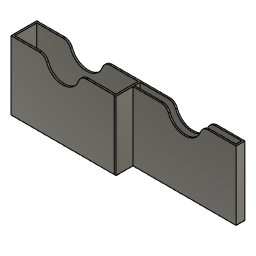
Food_Chain_Magnate_Reserve_CEO v1 (Autodesk Fusion 360 design; units mm, degrees)
Autodesk Fusion 360 part; units mm, degrees
sketch "Sketch1" plane through (0, 0, 0) normal (0, 0, 1) x (1, 0, 0)
  line L0 (-48.6499, 24.8) -> (41.3501, 24.8)
  line L1 (40, 23.2) -> (40, 3.6)
  line L2 (40, 2) -> (-51.6764, 2)
  line L3 (-50, 3.6) -> (-50, 23.2)
  line L4 (-51.6, 24.7889) -> (-51.6, 2)
  line L5 (-51.6, 2) -> (-51.6764, 2)
  line L6 (-51.6, 24.7889) -> (-48.6499, 24.8)
  line L7 (41.3501, 24.8) -> (41.6, 24.8)
  line L8 (41.6, 2) -> (40, 2)
  line L9 (-50, 23.2) -> (40, 23.2)
  line L10 (-50, 3.6) -> (40, 3.6)
  line L11 (41.6, 17) -> (131.6, 17)
  line L12 (41.6, 18.4) -> (131.6, 18.4)
  line L13 (41.6, 24.8) -> (131.6, 24.8)
  line L14 (41.6, 23.4) -> (131.6, 23.4)
  line L15 (131.6, 18.4) -> (131.6, 23.4)
  line L16 (131.6, 24.8) -> (133.2, 24.8)
  line L17 (131.6, 17) -> (133.2, 17)
  line L18 (133.2, 17) -> (133.2, 24.8)
  line L19 (41.6, 23.4) -> (41.6, 18.4)
  line L20 (41.6, 17) -> (41.6, 2)
  dimension "d1" = 90
  dimension "d2" = 23
  dimension "d3" = 1.6
  dimension "d4" = 1.6
  dimension "d5" = 1.6
  dimension "d6" = 1.6
  dimension "d7" = 90
  dimension "d8" = 15
  dimension "d9" = 90
  dimension "d10" = 1.4
  dimension "d11" = 90
  dimension "d12" = 90
  dimension "d13" = 90
  dimension "d14" = 1.4
  dimension "d15" = 1.6
  dimension "d16" = 1.6
  constraint horizontal L0
  constraint vertical L1
  constraint horizontal L2
  constraint vertical L3
  constraint vertical L4
  constraint perpendicular L1 L7
  constraint perpendicular L7 L19
  constraint perpendicular L1 L9
  constraint perpendicular L3 L10
  constraint coincident L11.start L19
  constraint perpendicular L11 L19
  constraint perpendicular L12 L19
  constraint perpendicular L13 L19
  constraint perpendicular L14 L19
  constraint perpendicular L14 L15
  constraint perpendicular L15 L16
  constraint parallel L11 L17
  constraint perpendicular L16 L18
  constraint collinear L19 L20
  measures "d1" distance of L0.start L0.end
  measures "d2" distance of L0.start L2.end
  measures "d3" distance of L1 L19
  measures "d4" distance of L3 L4
  measures "d5" distance of L2 L10
  measures "d6" distance of L0 L9
  measures "d7" distance of L11.start L11.end
  measures "d8" distance of L8.start L11
  measures "d9" distance of L12.start L12.end
  measures "d10" distance of L11 L12
  measures "d11" distance of L7.end L13.end
  measures "d12" distance of L14.start L14.end
  measures "d13" distance of L7.end L13.end
  measures "d14" distance of L13 L14
  measures "d15" distance of L13.end L16.end
  measures "d16" distance of L11.end L17.end
extrude "Extrude1" add sketch "Sketch1" along normal blind 61
extrude "Extrude2" add sketch "Sketch1" along normal blind 1 contours L1 L3 L9 L10 | L12 L14 L15 L19
sketch "Sketch2" plane through (0, 2, 0) normal (0, -1, 0) x (1, 0, 0)
  line L0 (-51.6, 0) -> (40, 0)
  line L1 (40, 0) -> (40, 61)
  line L2 (40, 61) -> (-51.6, 61)
  line L3 (-51.6, 61) -> (-51.6, 0)
  arc A0 (-20.8, 61) -> (9.2, 61) centre (-5.8, 61) ccw
  dimension "d21" = 30
  constraint midpoint L2 A0.centre
  constraint coincident L2 A0.end
  constraint coincident L2 A0.start
  measures "d21" diameter of A0
sketch "Sketch3" plane through (0, 17, 0) normal (0, -1, 0) x (1, 0, 0)
  line L0 (41.6, 0) -> (133.2, 0)
  line L1 (133.2, 0) -> (133.2, 61)
  line L2 (133.2, 61) -> (41.6, 61)
  line L3 (41.6, 61) -> (41.6, 0)
  arc A0 (72.4, 61) -> (102.4, 61) centre (87.4, 61) ccw
  dimension "d22" = 30
  constraint midpoint L2 A0.centre
  constraint coincident L2 A0.end
  constraint coincident L2 A0.start
  measures "d22" diameter of A0
extrude "Extrude3" cut sketch "Sketch2" against normal blind 41 contours L2 A0
extrude "Extrude4" cut sketch "Sketch3" against normal blind 28 contours L2 A0
fillet "Fillet1" radius 7 8 edges at (-20.8, 24, 61) (-20.8, 2.8, 61) (9.2, 2.8, 61) (9.2, 24, 61) (72.4, 24.1, 61) (72.4, 17.7, 61) (102.4, 17.7, 61) (102.4, 24.1, 61)
